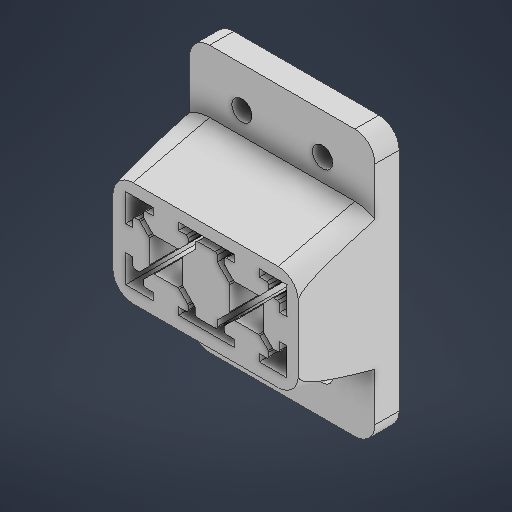
# Autodesk Inventor part: vslot_holder
Saved by Autodesk Inventor 2026.1 (Build 301233020, 233B)
## iProperties
Created: 2025-12-18
Part Number: vslot_holder
Material: Ogólny
Document SubType Name: Modeling
Designer: maciej
Density: 1 g/cm^3
Appearance: Domyślna
Author: maciej
Autodesk Inventor part; units mm, degrees
ref_plane "YZ Plane" through (0, 0, 0) normal (1, 0, 0) x (0, 1, 0)
ref_plane "XZ Plane" through (0, 0, 0) normal (0, 1, 0) x (-1, 0, 0)
ref_plane "XY Plane" through (0, 0, 0) normal (0, 0, 1) x (1, 0, 0)
sketch "Sketch1" plane through (0, 0, 0) normal (0, 0, 1) x (1, 0, 0)
  line L0 (4.1857, -4.1857) -> (4.1857, 4.1857)
  line L1 (-4.1857, -4.1857) -> (4.1857, -4.1857)
  line L2 (-3.125, -8.2) -> (-4.925, -10)
  line L3 (-10, -8.2) -> (10, -8.2)
  line L4 (10, 10) -> (10, -10)
  line L5 (10, -10) -> (-10, -10)
  line L6 (-10, 8.2) -> (10, 8.2)
  line L7 (-10, 10) -> (10, 10)
  line L8 (10, -10) -> (-10, 10) construction
  line L9 (-10, -10) -> (10, 10) construction
  line L10 (-8.2, 10) -> (-8.2, -10)
  line L11 (-10, -10) -> (-10, 10)
  line L12 (4.1857, -3.125) -> (7.3007, -6.24)
  line L13 (-7.1393, -8.2) -> (-3.125, -4.1857)
  line L14 (7.3007, -6.24) -> (7.3007, -8.2)
  line L15 (3.125, -8.2) -> (4.925, -10)
  circle A0 centre (0, 0) radius 2.1
  line L16 (10, -10) -> (10, 10)
  line L17 (30, -10) -> (10, -10)
  line L18 (30, 10) -> (30, -10)
  line L19 (10, 10) -> (30, 10)
  line L20 (-4.925, 10) -> (-3.125, 8.2)
  line L21 (-7.1393, 8.2) -> (-3.125, 4.1857)
  line L22 (-8.2, 7.1393) -> (-4.1857, 3.125)
  line L23 (-8.2, 5.4993) -> (-6.56, 5.4993)
  line L24 (-8.2, 3.125) -> (-10, 4.925)
  line L25 (-5.4993, 8.2) -> (-5.4993, 6.56)
  line L26 (4.1857, 4.1857) -> (-4.1857, 4.1857)
  line L27 (4.925, 10) -> (3.125, 8.2)
  line L28 (5.4993, 8.2) -> (5.4993, 6.56)
  line L29 (3.125, 4.1857) -> (7.1393, 8.2)
  line L30 (7.3007, 6.24) -> (7.3007, 8.2)
  line L31 (4.1857, 3.125) -> (7.3007, 6.24)
  line L32 (-4.1857, 4.1857) -> (-4.1857, -4.1857)
  line L33 (-8.2, -7.1393) -> (-4.1857, -3.125)
  line L34 (-8.2, -5.4993) -> (-6.56, -5.4993)
  line L35 (-5.4993, -6.56) -> (-5.4993, -8.2)
  line L36 (-8.2, -3.125) -> (-10, -4.925)
  line L37 (5.4993, -6.56) -> (5.4993, -8.2)
  line L38 (3.125, -4.1857) -> (7.1393, -8.2)
  line L39 (15.8143, 4.1857) -> (24.1857, 4.1857)
  line L40 (24.1857, 4.1857) -> (24.1857, -4.1857)
  line L41 (24.1857, -4.1857) -> (15.8143, -4.1857)
  line L42 (15.8143, -4.1857) -> (15.8143, 4.1857)
  line L43 (15.8143, -3.125) -> (12.6993, -6.24)
  line L44 (16.875, -4.1857) -> (12.8607, -8.2)
  line L45 (14.5007, -6.56) -> (14.5007, -8.2)
  line L46 (30, -8.2) -> (10, -8.2)
  line L47 (12.6993, -6.24) -> (12.6993, -8.2)
  line L48 (16.875, -8.2) -> (15.075, -10)
  line L49 (23.125, -8.2) -> (24.925, -10)
  line L50 (28.2, 10) -> (28.2, -10)
  line L51 (28.2, -7.1393) -> (24.1857, -3.125)
  line L52 (27.1393, -8.2) -> (23.125, -4.1857)
  line L53 (25.4993, -6.56) -> (25.4993, -8.2)
  line L54 (28.2, -5.4993) -> (26.56, -5.4993)
  line L55 (28.2, -3.125) -> (30, -4.925)
  line L56 (28.2, 3.125) -> (30, 4.925)
  line L57 (28.2, 5.4993) -> (26.56, 5.4993)
  line L58 (28.2, 7.1393) -> (24.1857, 3.125)
  line L59 (27.1393, 8.2) -> (23.125, 4.1857)
  line L60 (30, 8.2) -> (10, 8.2)
  line L61 (24.925, 10) -> (23.125, 8.2)
  line L62 (15.075, 10) -> (16.875, 8.2)
  line L63 (16.875, 4.1857) -> (12.8607, 8.2)
  line L64 (14.5007, 8.2) -> (14.5007, 6.56)
  line L65 (12.6993, 6.24) -> (12.6993, 8.2)
  line L66 (15.8143, 3.125) -> (12.6993, 6.24)
  circle A1 centre (20, 0) radius 2.1
  line L67 (-13, 13) -> (33, 13)
  line L68 (33, 13) -> (33, -13)
  line L69 (33, -13) -> (-13, -13)
  line L70 (-13, -13) -> (-13, 13)
  line L71 (-10, -8.2) -> (-13, -8.2)
  line L72 (30, -8.2) -> (33, -8.2)
  line L73 (-3.125, 8.2) -> (-3.125, 10)
  line L74 (3.125, 8.2) -> (3.125, 10)
  line L75 (-8.2, 3.125) -> (-10, 3.125)
  line L76 (-8.2, -3.125) -> (-10, -3.125)
  line L77 (-3.125, -8.2) -> (-3.125, -10)
  line L78 (3.125, -8.2) -> (3.125, -10)
  line L79 (16.875, -8.2) -> (16.875, -10)
  line L80 (23.125, -8.2) -> (23.125, -10)
  line L81 (28.2, -3.125) -> (30, -3.125)
  line L82 (28.2, 3.125) -> (30, 3.125)
  line L83 (23.125, 8.2) -> (23.125, 10)
  line L84 (16.875, 8.2) -> (16.875, 10)
  line L85 (-10, 10) -> (-10, 13)
  line L86 (10, 10) -> (10, 13)
  line L87 (14.5007, 8.2) -> (14.5007, 6.56)
  line L88 (14.5007, 8.2) -> (14.5007, 6.56)
  line L89 (25.4993, 6.56) -> (25.4993, 8.2)
  point P0 (0, 0)
  point P1 (0, 0)
  point P2 (0, -8.2)
  point P3 (0, 0)
  dimension "d0" = 4.2
  dimension "d1" = 20
  dimension "d2" = 1.8
  dimension "d3" = 20
  dimension "d4" = 20
  dimension "d5" = 1.8
  dimension "d6" = 1.8
  dimension "d7" = 1.5
  dimension "d8" = 0.75
  dimension "d9" = 135
  dimension "d10" = 6.25
  dimension "d11" = 3.125
  dimension "d12" = 1.5
  dimension "d13" = 1.5
  dimension "d14" = 1.5
  dimension "d15" = 0.75
  dimension "d16" = 0.75
  dimension "d17" = 0.75
  dimension "d18" = 1.64
  dimension "d19" = 1.64
  dimension "d20" = 1.64
  dimension "d21" = 1.64
  dimension "d22" = 1.64
  dimension "d23" = 1.64
  dimension "d24" = 45
  dimension "d25" = 1.96
  dimension "d26" = 1.96
  dimension "d27" = 3
  dimension "d28" = 3
  dimension "d29" = 3
  dimension "d30" = 3
  constraints: 172 end point, 75 point on line, 49 symmetric about line, 24 perpendicular, 13 parallel, 9 vertical, 5 horizontal, 4 coincident, 4 vertical alignment, 3 midpoint, 2 centre point, 2 horizontal alignment, 42 other
  measures "d0" diameter of A0
  measures "d1" distance of L85.start L86.start
  measures "d2" distance between parallel lines of L11 L10
  measures "d3" distance of L18.start L17.start
  measures "d4" distance between parallel lines of L18 L4
  measures "d7" distance between parallel lines of L21 L22
  measures "d8" distance between parallel lines of L21 L8
  measures "d9" angle of L7 L20
  measures "d10" distance of L15.start L2.start
  measures "d11" distance of L2.start point (0, -8.2)
  measures "d12" distance between parallel lines of L31 L29
  measures "d13" distance between parallel lines of L12 L38
  measures "d14" distance between parallel lines of L33 L13
  measures "d15" distance between parallel lines of L13 L9
  measures "d16" distance between parallel lines of L8 L12
  measures "d17" distance between parallel lines of L29 L9
  measures "d18" distance of L25.start L25.end
  measures "d19" distance of L23.start L23.end
  measures "d20" distance of L35.start L35.end
  measures "d21" distance of L34.start L34.end
  measures "d22" distance of L37.start L37.end
  measures "d23" distance of L28.start L28.end
  measures "d24" angle of L10 L24
  measures "d25" distance of L30.start L30.end
  measures "d26" distance of L12.end L14.end
  measures "d27" distance between parallel lines of L67 L7
  measures "d28" distance between parallel lines of L69 L5
  measures "d29" distance between parallel lines of L70 L11
  measures "d30" distance between parallel lines of L68 L18
extrude "Extrusion1" add sketch "Sketch1" along normal blind 20 contours L0 L31 L30 L6 L4 L3 L14 L12 | L38 L37 L3 L35 L13 L1 | L26 L21 L25 L6 L28 L29 | L4 L60 L65 L66 L42 L43 L47 L46 | L33 L34 L10 L23 L22 L32 | L78 L5 L77 L3 | L17 L18 L72 L68 L69 L70 L71 L11 L5 | L86 L67 L68 L72 L18 L19 | L7 L85 L67 L86 | L71 L70 L67 L85 L11 | L6 L73 L7 L74 | L79 L46 L80 L17 | L46 L45 L44 L41 L52 L53 | L76 L11 L75 L10 | L19 L83 L60 L84 | L60 L89 L59 L39 L63 L64 | L40 L58 L57 L50 L54 L51 | L81 L50 L82 L18
extrude "Extrusion2" add sketch "Sketch1" against normal blind 5 contours L1 L32 L26 L0 | L0 L12 L14 L3 L38 L1 | L0 L31 L30 L6 L4 L3 L14 L12 | L38 L37 L3 L35 L13 L1 | L0 L26 L29 L6 L30 L31 | L13 L3 L10 L33 L32 L1 | L38 L3 L37 | L3 L4 L5 L15 | L35 L3 L13 | L26 L21 L25 L6 L28 L29 | L6 L27 L7 L4 | L46 L48 L17 L4 | L4 L60 L65 L66 L42 L43 L47 L46 | L33 L34 L10 L23 L22 L32 | L3 L2 L5 L10 | L78 L5 L77 L3 | L15 L5 L78 | L26 L32 L22 L10 L6 L21 | L28 L6 L29 | L4 L19 L62 L60 | L17 L18 L72 L68 L69 L70 L71 L11 L5 | L47 L43 L42 L41 L44 L46 | L33 L10 L34 | L10 L5 L11 L3 | L3 L11 L36 L10 | L77 L5 L2 | L21 L6 L25 | L86 L67 L68 L72 L18 L19 | L7 L85 L67 L86 | L60 L63 L39 L42 L66 L65 | L48 L79 L17 | L44 L45 L46 | L23 L10 L22 | L71 L70 L67 L85 L11 | L6 L10 L7 L20 | L74 L7 L27 | L6 L73 L7 L74 | L19 L84 L62 | L60 L64 L63 | L79 L46 L80 L17 | L46 L45 L44 L41 L52 L53 | L42 L39 L40 L41 | L10 L24 L11 L6 | L76 L11 L75 L10 | L36 L11 L76 | L6 L11 L7 L10 | L20 L7 L73 | L19 L83 L60 L84 | L60 L89 L59 L39 L63 L64 | L80 L49 L17 | L46 L50 L17 L49 | L75 L11 L24 | L19 L61 L83 | L61 L19 L50 L60 | L53 L52 L46 | L41 L40 L51 L50 L46 L52 | L60 L59 L89 | L46 L50 L55 L18 | L18 L17 L50 L46 | L59 L60 L50 L58 L40 L39 | L19 L18 L60 L50 | L55 L81 L18 | L40 L58 L57 L50 L54 L51 | L60 L18 L56 L50 | L81 L50 L82 L18 | L51 L54 L50 | L50 L57 L58 | L82 L56 L18 | A0 | A1
move faces "Move1" translate (0.1768, 0.1768, 0) faces at (-4.9771, 3.9164, 6.6667) (-4.1857, -1.0417, 6.6667) (-7.1067, 5.4993, 13.3333) (-8.8, 3.125, 6.6667) (-10, 5.4167, 6.6667) (-3.9164, 8.2, 13.3333) (4.7079, 8.2, 13.3333) (3.125, 8.8, 6.6667) (10.8998, 8.2, 6.6667) (12.6993, 6.8933, 6.6667) (14.776, 4.1633, 6.6667) (15.8143, -1.0417, 6.6667) (12.6993, -7.5467, 6.6667) (1.0417, -4.1857, 6.6667) (4.7079, -5.7686, 13.3333) (5.4993, -7.6533, 6.6667) (-1.0417, 4.1857, 6.6667) (-4.7079, 5.7686, 6.6667) (-5.4993, 7.6533, 6.6667) (-8.2, 4.7079, 6.6667) (-3.125, 9.4, 6.6667) (-7.7083, 10, 6.6667) (7.7083, 10, 6.6667) (3.9164, 4.9771, 13.3333) (7.3007, 7.5467, 6.6667) (6.2623, 5.2017, 6.6667) (4.1857, 1.0417, 6.6667) (5.224, -4.1633, 13.3333) (7.3007, -6.8933, 13.3333) (9.1002, -8.2, 6.6667) (-3.125, -8.8, 6.6667) (-4.7079, -8.2, 6.6667) (-5.4993, -7.1067, 6.6667) (-3.9164, -4.9771, 13.3333) (-7.6533, -5.4993, 6.6667) (-8.2, -3.9164, 6.6667) (-9.4, -3.125, 6.6667) (-10, -7.7083, 6.6667) (-5.4167, -10, 6.6667) (12.2917, -10, 6.6667) (3.125, -9.4, 6.6667) (16.875, -8.8, 6.6667) (15.2921, -8.2, 13.3333) (14.5007, -7.1067, 6.6667) (13.7377, -5.2017, 13.3333) (16.0836, -4.9771, 13.3333) (21.0417, -4.1857, 6.6667) (24.7079, -5.7686, 13.3333) (3.9164, -8.2, 13.3333) (-5.7686, -4.7079, 6.6667) (5.4993, 7.1067, 6.6667) (25.4993, -7.6533, 6.6667) (23.9164, -8.2, 6.6667) (23.125, -9.4, 6.6667) (27.7083, -10, 6.6667) (30, -5.4167, 6.6667) (24.9771, -3.9164, 6.6667) (17.6667, 4.3333, -5) (24.1857, 1.0417, 6.6667) (25.7686, 4.7079, 6.6667) (30, 7.7083, 6.6667) (25.4167, 10, 6.6667) (23.9164, 4.9771, 6.6667) (18.9583, 4.1857, 6.6667) (15.2921, 5.7686, 6.6667) (14.5007, 7.6533, 6.6667) (16.0836, 8.2, 13.3333) (16.875, 9.4, 6.6667) (23.125, 8.8, 6.6667) (24.7079, 8.2, 6.6667) (29.4, 3.125, 6.6667) (28.2, 3.9164, 6.6667) (27.6533, 5.4993, 13.3333) (28.8, -3.125, 6.6667) (28.2, -4.7079, 6.6667) (27.1067, -5.4993, 13.3333) (25.4993, 7.1067, 6.6667)
fillet "Fillet1" radius 0.5 44 edges at (-8.0232, -5.3226, 10) (-6.3832, -5.3226, 10) (-4.0089, -2.9482, 10) (-4.0089, 3.3018, 10) (-6.3832, 5.6761, 10) (-8.0232, 5.6761, 10) (-5.3226, 6.7368, 10) (-5.3226, 8.3768, 10) (-2.9482, 4.3624, 10) (3.3018, 4.3624, 10) (5.6761, 6.7368, 10) (5.6761, 8.3768, 10) (7.4774, 8.3768, 10) (12.8761, 8.3768, 10) (15.9911, 3.3018, 10) (15.9911, -2.9482, 10) (12.8761, -8.0232, 10) (7.4774, -8.0232, 10) (5.6761, -8.0232, 10) (5.6761, -6.3832, 10) (-5.3226, -8.0232, 10) (-5.3226, -6.3832, 10) (-2.9482, -4.0089, 10) (3.3018, -4.0089, 10) (4.3624, -2.9482, 10) (4.3624, 3.3018, 10) (14.6774, 6.7368, 10) (17.0518, 4.3624, 10) (23.3018, 4.3624, 10) (14.6774, 8.3768, 10) (25.6761, 6.7368, 10) (25.6761, 8.3768, 10) (28.3768, 5.6761, 10) (26.7368, 5.6761, 10) (24.3624, 3.3018, 10) (24.3624, -2.9482, 10) (26.7368, -5.3226, 10) (28.3768, -5.3226, 10) (17.0518, -4.0089, 10) (23.3018, -4.0089, 10) (14.6774, -6.3832, 10) (14.6774, -8.0232, 10) (25.6761, -6.3832, 10) (25.6761, -8.0232, 10)
fillet "Fillet2" radius 5 4 edges at (-13, 13, 7.5) (33, 13, 7.5) (-13, -13, 7.5) (33, -13, 7.5)
sketch "Sketch2" plane through (28, -13, -5) normal (0, 0, -1) x (-1, 0, 0)
  arc A0 (-5, 5) -> (0, 0) centre (0, 5) ccw projected
  line L0 (0, 0) -> (36, 0) projected
  arc A1 (36, 0) -> (41, 5) centre (36, 5) ccw projected
  line L1 (41, 5) -> (41, 21) projected
  arc A2 (41, 21) -> (36, 26) centre (36, 21) ccw projected
  line L2 (36, 26) -> (0, 26) projected
  arc A3 (0, 26) -> (-5, 21) centre (0, 21) ccw projected
  line L3 (-5, 21) -> (-5, 5) projected
  line L4 (0, 0) -> (-5, 0)
  line L5 (-5, 0) -> (-5, 5)
  line L6 (36, 0) -> (41, 0)
  line L7 (41, 0) -> (41, 5)
  line L8 (0, 26) -> (-5, 26)
  arc A4 (0, 26) -> (-5, 21) centre (0, 21) ccw projected
  line L9 (-5, 26) -> (-5, 21)
  line L10 (41, 21) -> (41, 26)
  line L11 (41, 26) -> (36, 26)
  line L12 (-5, 0) -> (41, 0)
  line L13 (41, 0) -> (41, -20)
  line L14 (41, -20) -> (-5, -20)
  line L15 (-5, -20) -> (-5, 0)
  line L16 (-5, 26) -> (41, 26)
  line L17 (41, 26) -> (41, 46)
  line L18 (41, 46) -> (-5, 46)
  line L19 (-5, 46) -> (-5, 26)
  circle A5 centre (8, 36) radius 2.5
  circle A6 centre (28, 36) radius 2.5
  circle A7 centre (8, -10) radius 2.5
  circle A8 centre (28, -10) radius 2.5
  point P0 (28, 13)
  point P1 (41, 0)
  dimension "d48" = 20
  dimension "d49" = 20
  dimension "d50" = 5
  dimension "d51" = 5
  dimension "d52" = 5
  dimension "d53" = 5
  dimension "d54" = 13
  dimension "d55" = 13
  dimension "d56" = 10
  dimension "d57" = 10
  dimension "d63" = 20
  dimension "d64" = 13
  constraints: 32 end point, 8 tangent, 5 perpendicular, 4 centre point, 4 horizontal, 4 parallel, 2 coincident, 2 collinear, 2 horizontal alignment, 1 vertical
  measures "d48" distance between parallel lines of L0 L14
  measures "d49" distance between parallel lines of L2 L18
  measures "d50" diameter of A5
  measures "d51" diameter of A6
  measures "d52" diameter of A7
  measures "d53" diameter of A8
  measures "d54" distance from line of L13 A8.centre
  measures "d55" distance from line of L15 A7.centre
  measures "d56" distance from line of L14 A7.centre
  measures "d57" distance from line of L2 A5.centre
  measures "d63" distance of A5.centre A6.centre
  measures "d64" distance from line of L17 A6.centre
extrude "Extrusion3" add sketch "Sketch2" against normal blind 6 contours A0 L4 L5 | L0 L6 L13 L14 L15 L4 | L9 L8 A3 | A1 L7 L6 | L8 L19 L18 L17 L11 L2 | L11 L10 A2
fillet "Fillet3" radius 5 4 edges at (33, 33, -2) (-13, 33, -2) (-13, -33, -2) (33, -33, -2)
chamfer "Chamfer1" distance 4.5 distance2 19 3 edges at (-11.5355, 11.5355, 1) (10, 13, 1) (31.5355, 11.5355, 1) measured on face at (31.8891, 11.8891, 1) measured on face at (-11.8891, 11.8891, 1) measured on face at (10, 13.5, 1)
chamfer "Chamfer2" distance 4.5 distance2 19 3 edges at (10, -13, 1) (31.5355, -11.5355, 1) (-11.5355, -11.5355, 1) measured on face at (31.8891, -11.8891, 1) measured on face at (10, -13.5, 1) measured on face at (-11.8891, -11.8891, 1)
body "Solid1"
